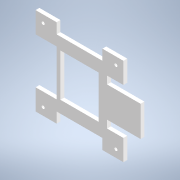
# Autodesk Inventor part: holder
Saved by Autodesk Inventor 2020 (Build 240168000, 168)
## iProperties
Created: 2019-06-13
Part Number: holder
Material: ABS Plastic
Document SubType Name: Modeling
Designer: amirt
Density: 1.06 g/cm^3
Appearance: Smooth - White
Author: amirt
Autodesk Inventor part; units mm, degrees
ref_plane "YZ Plane" through (0, 0, 0) normal (1, 0, 0) x (0, 1, 0)
ref_plane "XZ Plane" through (0, 0, 0) normal (0, 1, 0) x (-1, 0, 0)
ref_plane "XY Plane" through (0, 0, 0) normal (0, 0, 1) x (1, 0, 0)
sketch "Sketch1" plane through (0, 0, 0) normal (0, 0, 1) x (1, 0, 0)
  circle A0 centre (24.2455, 24.2455) radius 1.016 projected
  circle A1 centre (-24.2455, 24.2455) radius 1.016 projected
  circle A2 centre (-24.2455, -24.2455) radius 1.016 projected
  circle A3 centre (24.2455, -24.2455) radius 1.016 projected
  line L0 (29.2352, 15.2652) -> (29.2352, 29.2352)
  line L1 (29.2352, 29.2352) -> (15.2652, 29.2352)
  line L2 (29.2352, -15.2652) -> (29.2352, -29.2352)
  line L3 (29.2352, -29.2352) -> (15.2652, -29.2352)
  line L4 (-15.2652, -15.2652) -> (-29.2352, -15.2652)
  line L5 (-29.2352, -15.2652) -> (-29.2352, -29.2352)
  line L6 (-29.2352, -29.2352) -> (-15.2652, -29.2352)
  line L7 (-15.2652, -29.2352) -> (-15.2652, -15.2652)
  line L8 (-15.2652, 15.2652) -> (-29.2352, 15.2652)
  line L9 (-29.2352, 15.2652) -> (-29.2352, 29.2352)
  line L10 (-29.2352, 29.2352) -> (-15.2652, 29.2352)
  line L11 (-15.2652, 29.2352) -> (-15.2652, 15.2652)
  line L12 (15.2652, 22.2502) -> (-15.2652, 22.2502)
  line L13 (-15.2652, 22.2502) -> (-15.2652, -22.2502)
  line L14 (-15.2652, -22.2502) -> (15.2652, -22.2502)
  line L15 (23.114, 10.16) -> (18.034, 10.16) projected
  line L16 (18.034, -10.16) -> (23.114, -10.16) projected
  line L17 (40.6652, 10.16) -> (40.6652, -10.16)
  line L18 (12.7, 1.524) -> (12.7, 14.224) projected
  line L19 (12.7, -1.524) -> (12.7, -14.224) projected
  line L20 (-12.7, 14.224) -> (-12.7, 1.524) projected
  line L21 (-12.7, -14.224) -> (-12.7, -1.524) projected
  line L22 (12.7, 14.224) -> (-12.7, 14.224) projected
  line L23 (12.7, -1.524) -> (12.7, -14.224) projected
  line L24 (-12.7, -1.524) -> (12.7, -1.524) projected
  line L25 (-12.7, -14.224) -> (-12.7, -1.524) projected
  line L26 (12.7, -14.224) -> (-12.7, -14.224) projected
  line L27 (12.7, 14.224) -> (-12.7, 14.224)
  line L28 (-12.7, 14.224) -> (-12.7, -14.224)
  line L29 (-12.7, -14.224) -> (12.7, -14.224)
  line L30 (12.7, -14.224) -> (12.7, 14.224)
  line L31 (24.1704, 18.3364) -> (18.3759, 24.1384) projected
  line L32 (18.3759, -22.2502) -> (15.2652, -22.2502)
  line L33 (15.2652, 22.2502) -> (18.3759, 22.2502)
  line L34 (15.2652, 29.2352) -> (15.2652, 22.2502)
  line L35 (15.2652, -29.2352) -> (15.2652, -22.2502)
  line L36 (29.2352, 15.2652) -> (18.3759, 15.2652)
  line L37 (29.2352, -15.2652) -> (18.3759, -15.2652)
  line L38 (40.6652, 10.16) -> (18.3759, 10.16)
  line L39 (40.6652, -10.16) -> (18.3759, -10.16)
  line L40 (23.3888, 7.874) -> (36.0888, 7.874)
  line L41 (36.0888, 7.874) -> (36.0888, -7.874)
  line L42 (36.0888, -7.874) -> (23.3888, -7.874)
  line L43 (23.3888, -7.874) -> (23.3888, 7.874)
  line L44 (18.3759, -15.2652) -> (18.3759, -10.16)
  line L45 (18.3759, 10.16) -> (18.3759, 15.2652)
  point P0 (0, 0)
  point P1 (-15.2652, 22.2502)
  dimension "d1" = 12.7
  dimension "d2" = 12.7
  dimension "d4" = 13.97
  dimension "d5" = 13.97
  dimension "d6" = 13.97
  dimension "d7" = 13.97
  dimension "d8" = 13.97
  dimension "d9" = 13.97
  dimension "d10" = 13.97
  dimension "d11" = 13.97
  dimension "d20" = 12.7
  dimension "d21" = 15.748
  constraints: 68 end point, 11 equal length, 5 horizontal, 5 perpendicular, 2 point on line, 2 vertical, 1 midpoint
  measures "d1" distance of A1.centre L8.start
  measures "d2" distance of A2.centre L4.start
  measures "d4" distance of L1.end L0.end
  measures "d5" distance of L0.end L0.start
  measures "d6" distance of L2.end L3.end
  measures "d7" distance of L2.start L2.end
  measures "d8" distance of L6.end L5.end
  measures "d9" distance of L5.end L4.end
  measures "d10" distance of L9.end L10.end
  measures "d11" distance of L8.end L9.end
  measures "d20" distance of L41.end L42.end
  measures "d21" distance of L40.end L41.end
extrude "Extrusion3" add sketch "Sketch1" along normal blind 2.54
body "Solid3"
